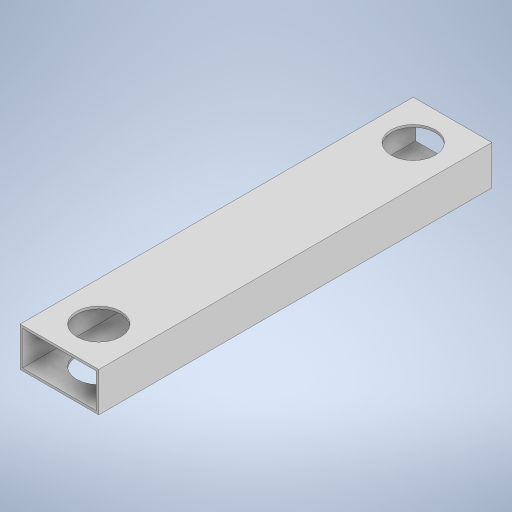
# Autodesk Inventor part: Main body
Saved by Autodesk Inventor 2023 (Build 270158000, 158)
## iProperties
Created: 2023-01-22
Part Number: Main body
Material: Generic
Document SubType Name: Modeling
Designer: matth
Density: 1 g/cm^3
Appearance: Default
Author: matth
Autodesk Inventor part; units mm, degrees
ref_plane "YZ Plane" through (0, 0, 0) normal (1, 0, 0) x (0, 1, 0)
ref_plane "XZ Plane" through (0, 0, 0) normal (0, 1, 0) x (-1, 0, 0)
ref_plane "XY Plane" through (0, 0, 0) normal (0, 0, 1) x (1, 0, 0)
sketch "Sketch1" plane through (0, 0, 0) normal (0, 0, 1) x (1, 0, 0)
  line L0 (0, 0) -> (50.8, 0)
  line L1 (50.8, 0) -> (50.8, 25.4)
  line L2 (50.8, 25.4) -> (0, 25.4)
  line L3 (0, 25.4) -> (0, 0)
  dimension "d0" = 50.8
  dimension "d1" = 25.4
  constraints: 8 end point, 2 parallel, 1 horizontal, 1 perpendicular
  measures "d0" distance of L2.end L1.end
  measures "d1" distance of L1.end L0.end
extrude "Extrusion1" add sketch "Sketch1" along normal blind 254
shell "Shell1" thickness 1.5875 removed faces 2 at (16.9333, 8.4667, 0) at (16.9333, 8.4667, 254)
sketch "Sketch2" plane through (0, 25.4, 0) normal (0, 1, 0) x (1, 0, 0)
  circle A0 centre (25.4, -25.4) radius 14.2875
  circle A1 centre (25.4, -228.6) radius 14.2875
  line L0 (0, -254) -> (50.8, -254) projected
  line L1 (50.8, 0) -> (0, 0) projected
  line L2 (0, 0) -> (0, -254) projected
  dimension "d5" = 25.4
  dimension "d6" = 25.4
  dimension "d7" = 25.4
  dimension "d8" = 25.4
  dimension "d9" = 28.575
  constraints: 2 centre point, 1 equal radius
  measures "d5" distance from line of L0 A1.centre
  measures "d6" distance from line of L1 A0.centre
  measures "d7" distance from line of L2 A0.centre
  measures "d8" distance from line of L2 A1.centre
  measures "d9" diameter of A1
extrude "Extrusion2" cut sketch "Sketch2" against normal through all
equation "\"d2\" = Length"
equation "\"d6\" = d5"
equation "\"d7\" = d6"
equation "\"d8\" = d5"
equation "\"Length\" = 254"
body "Solid1"
